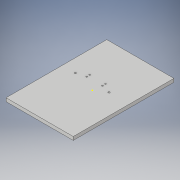
# Autodesk Inventor part: basestand
Saved by Autodesk Inventor 2019 (Build 230136000, 136)
## iProperties
Created: 2020-02-26
Part Number: basestand
Material: Generic
Document SubType Name: Modeling
Designer: Hp
Density: 1 g/cm^3
Appearance: Default
Author: Hp
Autodesk Inventor part; units mm, degrees
ref_plane "YZ Plane" through (0, 0, 0) normal (1, 0, 0) x (0, 1, 0)
ref_plane "XZ Plane" through (0, 0, 0) normal (0, 1, 0) x (-1, 0, 0)
ref_plane "XY Plane" through (0, 0, 0) normal (0, 0, 1) x (1, 0, 0)
sketch "Sketch1" plane through (0, 0, 0) normal (0, 1, 0) x (-1, 0, 0)
  line L0 (109.7414, 147.3061) -> (-90.2586, 147.3061)
  line L1 (-90.2586, 147.3061) -> (-90.2586, -152.6939)
  line L2 (-90.2586, -152.6939) -> (109.7414, -152.6939)
  line L3 (109.7414, -152.6939) -> (109.7414, 147.3061)
  circle A0 centre (70.1988, -19.7764) radius 2.5
  circle A1 centre (-29.8012, -19.7764) radius 2.5
  line L4 (70.1988, -19.7764) -> (-29.8012, -19.7764)
  point P0 (0, 0)
  dimension "d0" = 200
  dimension "d1" = 300
  dimension "d2" = 5
  dimension "d3" = 5
  dimension "d4" = 100
  constraints: 10 end point, 2 centre point, 2 horizontal, 2 parallel, 1 coincident, 1 perpendicular
  measures "d0" distance of L2.end L1.end
  measures "d1" distance of L1.end L0.end
  measures "d2" diameter of A0
  measures "d3" diameter of A1
  measures "d4" distance of L4.start L4.end
extrude "Extrusion1" add sketch "Sketch1" along normal blind 10
sketch "Sketch3" plane through (0, 10, 0) normal (0, 1, 0) x (1, 0, 0)
  point P0 (0, 0)
sketch "Sketch4" plane through (0, 10, 0) normal (0, 1, 0) x (1, 0, 0)
  circle A0 centre (-44.2796, 27.4201) radius 2
  circle A1 centre (2.7183, 27.4201) radius 2
  circle A2 centre (-44.2796, 36.422) radius 2
  circle A3 centre (2.7183, 36.422) radius 2
  point P0 (0, 0)
  dimension "d11" = 4
  dimension "d13" = 4
  dimension "d16" = 4
  dimension "d17" = 4
  constraints: 4 centre point
  measures "d11" diameter of A0
  measures "d13" diameter of A1
  measures "d16" diameter of A2
  measures "d17" diameter of A3
extrude "Extrusion3" cut sketch "Sketch4" against normal blind 10
body "Solid1"
